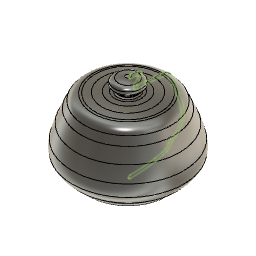
Week 3 HW Teapot Drawing (Autodesk Fusion 360 archive; units mm, degrees)
design "Week 3 HW Teapot"
Autodesk Fusion 360 part; units mm, degrees
sketch "Sketch5" plane through (0, 0, 0) normal (1, 0, 0) x (0, 1, 0)
  spline S0 degree 3 poles (3.9161, 150.5174) (2.5137, 150.5885) (1.3191, 149.5092) (1.2481, 148.1067) knots 0 0 0 0 1 1 1 1
  spline S1 degree 3 poles (1.2481, 148.1067) (1.177, 146.7042) (2.2563, 145.5097) (3.6588, 145.4386) knots 0 0 0 0 1 1 1 1
  spline S2 degree 2 poles (3.6588, 145.4386) (10.0259, 145.0651) (14.4674, 143.6904) knots 0 0 0 1 1 1
  spline S3 degree 3 poles (14.4674, 143.6904) (16.6882, 143.0031) (18.1122, 141.858) (18.1726, 141.7298) knots 0 0 0 0 1 1 1 1
  spline S4 degree 3 poles (18.1726, 141.7298) (18.2029, 141.6657) (18.2785, 141.8339) (18.0682, 141.4089) knots 0 0 0 0 1 1 1 1
  spline S5 degree 3 poles (18.0682, 141.4089) (17.858, 140.984) (17.1856, 140.1195) (15.8224, 139.0592) knots 0 0 0 0 1 1 1 1
  spline S6 degree 3 poles (15.8224, 139.0592) (12.5526, 136.516) (10.6299, 134.4536) (9.7674, 132.1407) knots 0 0 0 0 1 1 1 1
  spline S7 degree 3 poles (9.7674, 132.1407) (9.3362, 130.9843) (9.2361, 129.6856) (9.6088, 128.5291) knots 0 0 0 0 1 1 1 1
  spline S8 degree 3 poles (9.6088, 128.5291) (9.9815, 127.3726) (10.7619, 126.4791) (11.5932, 125.8672) knots 0 0 0 0 1 1 1 1
  spline S9 degree 3 poles (11.5932, 125.8672) (13.2557, 124.6434) (15.1791, 124.2208) (17.1024, 123.9862) knots 0 0 0 0 1 1 1 1
  spline S10 degree 3 poles (17.1024, 123.9862) (19.0257, 123.7516) (20.9493, 123.7816) (22.5687, 123.9841) knots 0 0 0 0 1 1 1 1
  spline S11 degree 3 poles (22.5687, 123.9841) (23.216, 124.0651) (26.4385, 124.0163) (30.1972, 123.7541) knots 0 0 0 0 1 1 1 1
  spline S12 degree 3 poles (30.1972, 123.7541) (33.9559, 123.4919) (38.5055, 123.0752) (42.8331, 122.6235) knots 0 0 0 0 1 1 1 1
  spline S13 degree 3 poles (42.8331, 122.6235) (47.6357, 122.4298) (56.3609, 120.8515) (58.3516, 120.4298) knots 0 0 0 0 1 1 1 1
  spline S14 degree 2 poles (58.3516, 120.4298) (65.4322, 119.4494) (67.5877, 113.7527) knots 0 0 0 1 1 1
  spline S15 degree 3 poles (67.5877, 113.7527) (68.394, 111.6217) (70.396, 107.4426) (72.9734, 101.7064) knots 0 0 0 0 1 1 1 1
  spline S16 degree 3 poles (72.9734, 101.7064) (75.5508, 95.9702) (78.6538, 88.8254) (81.4535, 81.3665) knots 0 0 0 0 1 1 1 1
  spline S17 degree 3 poles (81.4535, 81.3665) (84.2532, 73.9077) (86.7464, 66.1281) (88.1125, 59.202) knots 0 0 0 0 1 1 1 1
  spline S18 degree 3 poles (88.1125, 59.202) (89.4787, 52.2759) (89.6189, 46.2085) (88.2407, 42.4268) knots 0 0 0 0 1 1 1 1
  spline S19 degree 3 poles (88.2407, 42.4268) (85.6934, 35.4372) (81.3176, 30.8464) (77.2315, 27.5305) knots 0 0 0 0 1 1 1 1
  spline S20 degree 3 poles (77.2315, 27.5305) (75.1885, 25.8726) (73.2286, 24.5507) (71.589, 23.399) knots 0 0 0 0 1 1 1 1
  spline S21 degree 3 poles (71.589, 23.399) (69.9494, 22.2473) (68.6038, 21.5199) (67.6099, 19.7858) knots 0 0 0 0 1 1 1 1
  spline S22 degree 3 poles (67.6099, 19.7858) (65.9871, 16.9544) (66.7776, 15.6324) (62.7203, 13.6306) knots 0 0 0 0 1 1 1 1
  spline S23 degree 3 poles (62.7203, 13.6306) (62.3503, 13.4481) (60.4071, 12.7076) (57.4943, 11.9026) knots 0 0 0 0 1 1 1 1
  spline S24 degree 3 poles (57.4943, 11.9026) (54.5814, 11.0976) (50.5698, 10.1489) (45.527, 9.2392) knots 0 0 0 0 1 1 1 1
  spline S25 degree 3 poles (45.527, 9.2392) (35.4416, 7.4196) (21.2285, 5.7526) (3.3342, 5.6554) knots 0 0 0 0 1 1 1 1
  spline S26 degree 3 poles (3.3342, 5.6554) (1.9299, 5.6479) (0.7976, 4.5033) (0.8052, 3.099) knots 0 0 0 0 1 1 1 1
  spline S27 degree 3 poles (0.8052, 3.099) (0.8127, 1.6946) (1.9573, 0.5623) (3.3616, 0.5699) knots 0 0 0 0 1 1 1 1
  spline S28 degree 3 poles (3.3616, 0.5699) (21.5569, 0.6688) (36.057, 2.3634) (46.4298, 4.2348) knots 0 0 0 0 1 1 1 1
  spline S29 degree 3 poles (46.4298, 4.2348) (51.6162, 5.1705) (55.7698, 6.15) (58.8492, 7.0011) knots 0 0 0 0 1 1 1 1
  spline S30 degree 3 poles (58.8492, 7.0011) (61.9286, 7.8521) (63.8043, 8.4949) (64.9703, 9.0702) knots 0 0 0 0 1 1 1 1
  spline S31 degree 3 poles (64.9703, 9.0702) (70.4789, 11.788) (71.4301, 16.224) (72.022, 17.2568) knots 0 0 0 0 1 1 1 1
  spline S32 degree 3 poles (72.022, 17.2568) (71.9234, 17.0846) (72.94, 18.133) (74.5123, 19.2375) knots 0 0 0 0 1 1 1 1
  spline S33 degree 3 poles (74.5123, 19.2375) (76.0847, 20.342) (78.1862, 21.7563) (80.436, 23.582) knots 0 0 0 0 1 1 1 1
  spline S34 degree 3 poles (80.436, 23.582) (84.9356, 27.2333) (90.0715, 32.5984) (93.0187, 40.6853) knots 0 0 0 0 1 1 1 1
  spline S35 degree 3 poles (93.0187, 40.6853) (94.9824, 46.0735) (94.5541, 52.821) (93.1014, 60.1859) knots 0 0 0 0 1 1 1 1
  spline S36 degree 3 poles (93.1014, 60.1859) (91.6487, 67.5508) (89.073, 75.5379) (86.2145, 83.1535) knots 0 0 0 0 1 1 1 1
  spline S37 degree 3 poles (86.2145, 83.1535) (83.3559, 90.7691) (80.2108, 98.0064) (77.6119, 103.7905) knots 0 0 0 0 1 1 1 1
  spline S38 degree 3 poles (77.6119, 103.7905) (75.013, 109.5746) (72.9106, 114.0545) (72.344, 115.552) knots 0 0 0 0 1 1 1 1
  spline S39 degree 3 poles (72.344, 115.552) (69.8713, 121.3085) (64.2092, 124.6033) (58.3521, 125.7649) knots 0 0 0 0 1 1 1 1
  spline S40 degree 3 poles (58.3521, 125.7649) (57.5105, 125.9328) (56.3346, 126.1151) (54.8495, 126.3214) knots 0 0 0 0 1 1 1 1
  spline S41 degree 3 poles (54.8495, 126.3214) (51.8792, 126.734) (47.7329, 127.2246) (43.3607, 127.681) knots 0 0 0 0 1 1 1 1
  spline S42 degree 3 poles (43.3607, 127.681) (38.9886, 128.1374) (34.3985, 128.5588) (30.5512, 128.8272) knots 0 0 0 0 1 1 1 1
  spline S43 degree 3 poles (30.5512, 128.8272) (26.7039, 129.0956) (23.8541, 129.2701) (21.9372, 129.0303) knots 0 0 0 0 1 1 1 1
  spline S44 degree 3 poles (21.9372, 129.0303) (20.7781, 128.8853) (19.1593, 128.8581) (17.7179, 129.0339) knots 0 0 0 0 1 1 1 1
  spline S45 degree 3 poles (17.7179, 129.0339) (16.2765, 129.2097) (15.0128, 129.6645) (14.608, 129.9625) knots 0 0 0 0 1 1 1 1
  spline S46 degree 3 poles (14.608, 129.9625) (14.4056, 130.1116) (14.4322, 130.1406) (14.4488, 130.0892) knots 0 0 0 0 1 1 1 1
  spline S47 degree 3 poles (14.4488, 130.0892) (14.4654, 130.0377) (14.4069, 130.0271) (14.5325, 130.3641) knots 0 0 0 0 1 1 1 1
  spline S48 degree 3 poles (14.5325, 130.3641) (14.7838, 131.038) (16.0361, 132.7832) (18.9447, 135.0454) knots 0 0 0 0 1 1 1 1
  spline S49 degree 3 poles (18.9447, 135.0454) (20.6706, 136.3878) (21.8905, 137.6672) (22.6261, 139.1537) knots 0 0 0 0 1 1 1 1
  spline S50 degree 3 poles (22.6261, 139.1537) (23.3617, 140.6403) (23.437, 142.4879) (22.7718, 143.8986) knots 0 0 0 0 1 1 1 1
  spline S51 degree 3 poles (22.7718, 143.8986) (21.4415, 146.72) (18.694, 147.7058) (15.9712, 148.5485) knots 0 0 0 0 1 1 1 1
  spline S52 degree 2 poles (15.9712, 148.5485) (10.5256, 150.234) (3.9161, 150.5174) knots 0 0 0 1 1 1
  line L0 (3.9161, 150.5174) -> (3.9161, 150.5174)
revolve "Revolve3" add sketch "Sketch5" angle 360 about axis through (0, 0, 1.75) along (0, 0, 1) contours S46 S47 | S0 S1 S2 S3 S4 S5 S6 S7 S8 S9 S10 S11 S12 S13 S14 S15 S16 S17 S18 S19 S20 S21 S22 S23 S24 S25 S26 S27 S28 S29 S30 S31 S32 S33 S34 S35 S36 S37 S38 S39 S40 S41 S42 S43 S44 S45 S46 S47 S48 S49 S50 S51 S52
